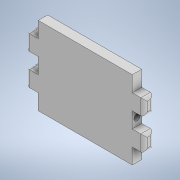
# Autodesk Inventor part: menteA
Saved by Autodesk Inventor 2020.2 (Build 242310000, 310)
## iProperties
Created: 2020-03-03
Part Number: menteA
Material: 一般
Document SubType Name: Modeling
Designer: touhu_zn72wdq
Density: 1 g/cm^3
Appearance: 既定
Author: touhu_zn72wdq
Autodesk Inventor part; units mm, degrees
ref_plane "YZ Plane" through (0, 0, 0) normal (1, 0, 0) x (0, 1, 0)
ref_plane "XZ Plane" through (0, 0, 0) normal (0, 1, 0) x (-1, 0, 0)
ref_plane "XY Plane" through (0, 0, 0) normal (0, 0, 1) x (1, 0, 0)
sketch "スケッチ1" plane through (0, 0, 0) normal (0, 0, 1) x (1, 0, 0)
  line L0 (0, 0) -> (75, 0)
  line L1 (75, 0) -> (75, 50)
  line L2 (75, 50) -> (0, 50)
  line L3 (0, 50) -> (0, 0)
  line L4 (0, 50) -> (7.5, 50)
  line L5 (7.5, 50) -> (7.5, 40)
  line L6 (7.5, 40) -> (0, 40)
  line L7 (0, 40) -> (0, 50)
  line L8 (75, 0) -> (0, 0)
  line L9 (0, 0) -> (0, 49.7722)
  line L10 (7.5, 0) -> (7.5, 10)
  line L11 (7.5, 10) -> (0, 10)
  line L12 (75, 0) -> (0, 0)
  line L13 (0, 50) -> (75, 50)
  line L14 (75, 50) -> (75, 0)
  line L15 (75, 50) -> (67.5, 50)
  line L16 (67.5, 50) -> (67.5, 40)
  line L17 (67.5, 40) -> (75, 40)
  line L18 (75, 40) -> (75, 50)
  line L19 (67.5, 0) -> (67.5, 10)
  line L20 (67.5, 10) -> (75, 10)
  line L21 (7.5, 30) -> (0, 30)
  line L22 (0, 30) -> (0, 20)
  line L23 (0, 20) -> (7.5, 20)
  line L24 (7.5, 20) -> (7.5, 30)
  line L25 (75, 50) -> (75, 0)
  line L26 (75, 0) -> (75, 49.7722)
  line L27 (67.5, 30) -> (75, 30)
  line L28 (75, 30) -> (75, 20)
  line L29 (75, 20) -> (67.5, 20)
  line L30 (67.5, 20) -> (67.5, 30)
  dimension "d0" = 75
  dimension "d1" = 50
  dimension "d2" = 7.5
  dimension "d3" = 10
  dimension "d4" = 10
  dimension "d5" = 10
  constraints: 62 end point, 6 parallel, 3 horizontal, 3 perpendicular, 2 point on line
  measures "d0" distance of L2.end L1.end
  measures "d1" distance of L1.end L0.end
  measures "d2" distance of L5.end L6.end
  measures "d3" distance of L4.end L5.end
  measures "d4" distance of L22.end L21.end
  measures "d5" distance between parallel lines of L21 L6
extrude "押し出し1" add sketch "スケッチ1" along normal blind 6 contours L10 L11 L3 L23 L24 L21 L6 L5 L2 L16 L17 L1 L27 L30 L29 L20 L19 L0
sketch "スケッチ2" plane through (7.5, 20, 0) normal (-1, 0, 0) x (0, 0, 1)
  line L0 (0, 10) -> (6, 10) projected
  line L1 (0, 10) -> (0, 0) projected
  point P0 (0, -20)
  point P1 (3, 5)
  dimension "d8" = 5
  dimension "d9" = 3
  measures "d8" distance from line of L0 point (3, 5)
  measures "d9" distance from line of L1 point (3, 5)
sketch "スケッチ3" plane through (67.5, 20, 0) normal (1, 0, 0) x (0, 0, -1)
  line L0 (-6, 0) -> (-6, 10) projected
  line L1 (0, 10) -> (-6, 10) projected
  point P0 (0, -20)
  point P1 (-3, 5)
  dimension "d10" = 3
  dimension "d11" = 5
  measures "d10" distance from line of L0 point (-3, 5)
  measures "d11" distance from line of L1 point (-3, 5)
hole "穴1" at (67.5, 25, 3) direction (-1, 0, 0) diameter 4 depth 4.5
hole "穴2" at (7.5, 25, 3) direction (1, 0, 0) diameter 4 depth 4.5
fillet "フィレット1" radius 2 16 edges at (75, 35, 0) (75, 35, 6) (75, 40, 3) (75, 30, 3) (75, 20, 3) (75, 15, 6) (75, 15, 0) (75, 10, 3) (0, 35, 0) (0, 40, 3) (0, 35, 6) (0, 30, 3) (0, 20, 3) (0, 15, 0) (0, 10, 3) (0, 15, 6)
